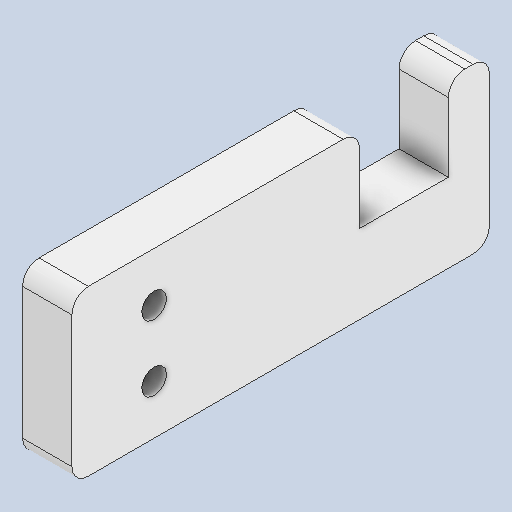
# Autodesk Inventor part: base_weel-v2-POM-pc-F-1
Saved by Autodesk Inventor 2025.2 (Build 292293000, 293)
## iProperties
Created: 2025-01-14
Part Number: base_weel-v2-POM-pc-F-1
Material: ABS プラスチック
Document SubType Name: Modeling
Designer: haruy
Density: 1.06 g/cm^3
Appearance: 白
Author: haruy
Autodesk Inventor part; units mm, degrees
ref_plane "YZ Plane" through (0, 0, 0) normal (1, 0, 0) x (0, 1, 0)
ref_plane "XZ Plane" through (0, 0, 0) normal (0, 1, 0) x (-1, 0, 0)
ref_plane "XY Plane" through (0, 0, 0) normal (0, 0, 1) x (1, 0, 0)
sketch "スケッチ1" plane through (0, 0, 0) normal (1, 0, 0) x (0, 1, 0)
  line L0 (0, 0) -> (20, 0)
  line L1 (20, 0) -> (20, -20)
  line L2 (20, -20) -> (0, -20)
  line L3 (0, -20) -> (0, 0)
  line L4 (102.9471, -35) -> (9.6, -35)
  line L5 (9.6, -35) -> (9.6, -45.8)
  line L6 (9.6, -45.8) -> (102.9471, -45.8)
  line L7 (102.9471, -45.8) -> (102.9471, -35)
  circle A0 centre (14, -10) radius 1.5
  circle A1 centre (6, -10) radius 1.5
  line L8 (20, -45.8) -> (0, -45.8)
  line L9 (0, -45.8) -> (0, -50.8)
  line L10 (0, -50.8) -> (20, -50.8)
  line L11 (20, -50.8) -> (20, -45.8)
  line L12 (0, -20) -> (0, -45.8)
  line L13 (20, -20) -> (20, -35)
  dimension "d0" = 20
  dimension "d1" = 20
  dimension "d2" = 10.8
  dimension "d3" = 9.6
  dimension "d4" = 15
  dimension "d5" = 3
  dimension "d6" = 3
  dimension "d7" = 10
  dimension "d8" = 10
  dimension "d9" = 6
  dimension "d10" = 8
  dimension "d11" = 5
  dimension "d12" = 20
  dimension "d13" = 0
  constraints: 28 end point, 6 parallel, 4 perpendicular, 3 horizontal, 2 centre point, 2 point on line
  measures "d0" distance of L0.end L1.end
  measures "d1" distance between parallel lines of L3 L1
  measures "d2" distance between parallel lines of L4 L6
  measures "d3" distance between parallel lines of L5 L3
  measures "d4" distance between parallel lines of L4 L2
  measures "d5" diameter of A0
  measures "d6" diameter of A1
  measures "d7" distance from line of A0.centre L0
  measures "d8" distance from line of A1.centre L0
  measures "d9" distance from line of A1.centre L3
  measures "d10" distance of A0.centre A1.centre
  measures "d11" distance between parallel lines of L6 L10
  measures "d12" distance between parallel lines of L9 L11
  measures "d13" distance between parallel lines of L3 L9
extrude "押し出し1" add sketch "スケッチ1" along normal blind 6 contours L0 L1 L2 L3 | L2 L13 L4 L5 L8 L12 | L8 L6 L11 L10 L9
fillet "フィレット1" radius 2 6 edges at (3, 0, 0) (3, 20, 0) (3, 20, -35) (3, 20, -45.8) (3, 20, -50.8) (3, 0, -50.8)
sketch "スケッチ2" plane through (6, 0, 0) normal (1, 0, 0) x (0, 0, -1)
  arc A0 (48.8, 0) -> (50.8, 2) centre (48.8, 2) ccw projected
  line L0 (50.8, 2) -> (50.8, 18) projected
  arc A1 (50.8, 18) -> (48.8, 20) centre (48.8, 18) ccw projected
  line L1 (48.8, 20) -> (47.8, 20) projected
  arc A2 (47.8, 20) -> (45.8, 18) centre (47.8, 18) ccw projected
  line L2 (45.8, 18) -> (45.8, 9.6) projected
  line L3 (45.8, 9.6) -> (35, 9.6) projected
  line L4 (35, 9.6) -> (35, 18) projected
  arc A3 (35, 18) -> (33, 20) centre (33, 18) ccw projected
  line L5 (33, 20) -> (2, 20) projected
  arc A4 (2, 20) -> (0, 18) centre (2, 18) ccw projected
  line L6 (0, 18) -> (0, 2) projected
  arc A5 (0, 2) -> (2, 0) centre (2, 2) ccw projected
  line L7 (2, 0) -> (48.8, 0) projected
  circle A6 centre (10, 6) radius 1.5 projected
  circle A7 centre (10, 14) radius 1.5 projected
  point P0 (0, 0)
equation "\"d12\" = d1"
